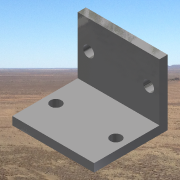
# Autodesk Inventor part: 0wrab
Saved by Autodesk Inventor 2013 SP2 (Build 170200200, 200)
## iProperties
Company: HERA Project
Created: 2013-12-30
Part Number: 0wrab
Material: Steel, Galvanized
Document SubType Name: Modeling
Designer: Dave
Density: 7.85 g/cm^3
Mass: 1047.5 g
Surface Area: 342.566 cm^2
Volume: 133.439 cm^3
Description: thick right angle for winch
Author: David DeBoer
Title: Thick Right Angle Bracket
Autodesk Inventor part; units mm, degrees
ref_plane "YZ Plane" through (0, 0, 0) normal (1, 0, 0) x (0, 1, 0)
ref_plane "XZ Plane" through (0, 0, 0) normal (0, 1, 0) x (-1, 0, 0)
ref_plane "XY Plane" through (0, 0, 0) normal (0, 0, 1) x (1, 0, 0)
sketch "Sketch1" plane through (0, 0, 0) normal (1, 0, 0) x (0, 1, 0)
  line L0 (0, 0) -> (76.2, 0)
  line L1 (76.2, 0) -> (76.2, 9.525)
  line L2 (76.2, 9.525) -> (9.525, 9.525)
  line L3 (0, 9.525) -> (0, 0)
  line L4 (9.525, 9.525) -> (9.525, 85.725)
  line L5 (9.525, 85.725) -> (0, 85.725)
  line L6 (0, 85.725) -> (0, 9.525)
  dimension "d4" = 76.2
  dimension "d5" = 9.525
  dimension "d6" = 9.525
  dimension "d7" = 76.2
  constraints: 14 end point, 3 parallel, 1 horizontal, 1 perpendicular
  measures "d4" distance of L5.end L3.start
  measures "d5" distance of L4.end L5.end
  measures "d6" distance of L3.start L0.start
  measures "d7" distance of L0.start L0.end
extrude "Extrusion1" add sketch "Sketch1" along normal blind 95.25
sketch "Sketch2" plane through (0, 9.525, 85.725) normal (0, 1, 0) x (1, 0, 0)
  line L0 (95.25, 76.2) -> (95.25, 0) projected
  circle A0 centre (82.55, 38.1) radius 4.4901
  circle A1 centre (12.7, 38.1) radius 5.7238
  point P0 (0, 85.725)
  dimension "d13" = 12.7
  dimension "d14" = 69.85
  constraints: 2 centre point
  measures "d13" distance from line of A0.centre L0
  measures "d14" distance of A1.centre A0.centre
hole "Hole1" at (12.7, 9.525, 47.625) at (82.55, 9.525, 47.625) direction (0, -1, 0) diameter 12.7 depth 25.4 tip angle 118
sketch "Sketch3" plane through (0, 9.525, 9.525) normal (0, 0, 1) x (1, 0, 0)
  line L0 (95.25, 66.675) -> (95.25, 0) projected
  circle A0 centre (82.55, 33.3375) radius 4.4901
  circle A1 centre (12.7, 33.3375) radius 3.5498
  point P0 (0, -9.525)
  dimension "d22" = 12.7
  dimension "d23" = 69.85
  constraints: 2 centre point
  measures "d22" distance from line of A0.centre L0
  measures "d23" distance of A1.centre A0.centre
hole "Hole2" at (12.7, 42.8625, 9.525) at (82.55, 42.8625, 9.525) direction (0, 0, -1) diameter 12.7 depth 25.4 tip angle 118
body "Solid1"
